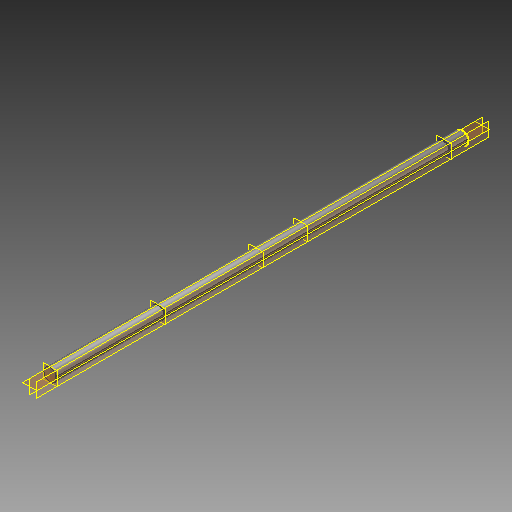
# Autodesk Inventor part: Pin .5in. Dia. - Boom Hinge
Saved by Autodesk Inventor 2019 (Build 230136000, 136)
## iProperties
Created: 2018-10-28
Part Number: Pin .5in. Dia. - Boom Hinge
Material: Stainless Steel
Document SubType Name: Modeling
Designer: Alex Barnett
Density: 8 g/cm^3
Appearance: Semi-Polished
Mass: 395.926 g
Surface Area: 176.218 cm^2
Volume: 49.4908 cm^3
Author: Alex Barnett
Autodesk Inventor part; units mm, degrees
sketch "Sketch1" plane through (0, 0, 0) normal (0, 0, 1) x (1, 0, 0)
  circle A0 centre (0, 0) radius 6.35
  dimension "d0" = 12.7
  constraints: 1 centre point, 1 coincident
  measures "d0" diameter of A0
extrude "Extrusion1" add sketch "Sketch1" along normal mid plane 406.4
ref_plane "Work Plane1" through (0, 0, 203.2) normal (0, 0, 1) x (1, 0, 0)
ref_plane "Work Plane2" through (0, 0, -185.7248) normal (0, 0, -1) x (-1, 0, 0)
sketch "Sketch2" plane through (0, 0, -185.7248) normal (0, 0, -1) x (-1, 0, 0)
  circle A0 centre (0, 0) radius 5.9436
  circle A1 centre (0, 0) radius 6.35
  dimension "d5" = 11.8872
  dimension "d6" = 12.7
  constraints: 2 centre point, 2 coincident
  measures "d5" diameter of A0
  measures "d6" diameter of A1
extrude "Extrusion2" cut sketch "Sketch2" against normal blind 0.9906
ref_plane "Work Plane3" through (0, 0, 96.8248) normal (0, 0, 1) x (1, 0, 0)
sketch "Sketch3" plane through (0, 0, 96.8248) normal (0, 0, 1) x (1, 0, 0)
  circle A0 centre (0, 0) radius 6.35
  circle A1 centre (0, 0) radius 5.9436
  dimension "d10" = 12.7
  dimension "d11" = 11.8872
  constraints: 2 centre point, 2 coincident
  measures "d10" diameter of A0
  measures "d11" diameter of A1
extrude "Extrusion3" cut sketch "Sketch3" against normal blind 0.9906
ref_plane "Work Plane4" through (6.35, 0, 0) normal (1, 0, 0) x (0, 1, 0)
sketch "Sketch5" plane through (0, 0, -203.2) normal (0, 0, -1) x (-1, 0, 0)
  circle A0 centre (0, 0) radius 6.35 projected
sketch "Sketch6" plane through (0, 0, -203.2) normal (0, 0, -1) x (-1, 0, 0)
  circle A0 centre (0, 0) radius 6.35 projected
  line L0 (-4.7625, -1.5875) -> (-7.9375, -1.5875)
  line L1 (-7.9375, -1.5875) -> (-7.9375, 1.5875)
  line L2 (-7.9375, 1.5875) -> (-4.7625, 1.5875)
  line L3 (-4.7625, 1.5875) -> (-4.7625, -1.5875)
  line L4 (-4.7625, -1.5875) -> (-7.9375, 1.5875) construction
  line L5 (-7.9375, -1.5875) -> (-4.7625, 1.5875) construction
  point P0 (-6.35, 0)
  dimension "d19" = 3.175
  dimension "d20" = 3.175
  constraints: 12 end point, 2 midpoint, 2 parallel, 1 horizontal, 1 horizontal alignment, 1 perpendicular, 1 other
  measures "d19" distance of L1.end L2.end
  measures "d20" distance of L0.end L1.end
extrude "Extrusion5" cut sketch "Sketch6" against normal blind 406.4 contours L2 L3 L0 A0 | A0 L0 L1 L2 picked at (-5.2842, -0.1781)
ref_plane "Midplane" through (0, 0, -44.45) normal (0, 0, 1) x (1, 0, 0)
body "Solid1"
